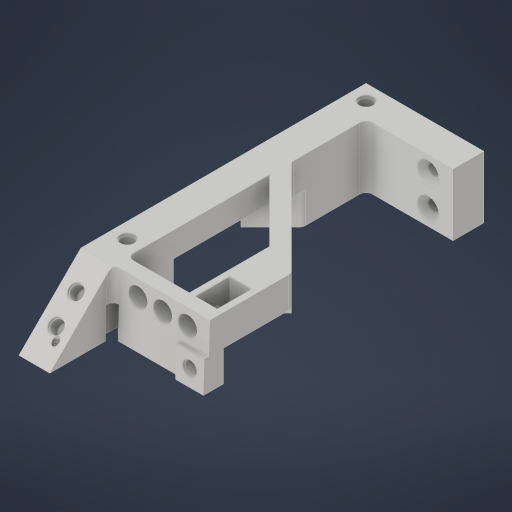
# Autodesk Inventor part: mocowanie-czujnika-p
Saved by Autodesk Inventor 2023 (Build 270158000, 158)
## iProperties
Created: 2019-09-07
Part Number: mocowanie-czujnika-p
Material: Generic
Document SubType Name: Modeling
Designer: Michal
Density: 1 g/cm^3
Appearance: Default
Author: Michal
Autodesk Inventor part; units mm, degrees
note: some values were not read from the file. Chosen so that the rebuilt part matches the saved one: direction of "Hole13".
ref_plane "YZ Plane" through (0, 0, 0) normal (1, 0, 0) x (0, 1, 0)
ref_plane "XZ Plane" through (0, 0, 0) normal (0, 1, 0) x (-1, 0, 0)
sketch "Sketch1" plane through (0, 0, 0) normal (1, 0, 0) x (0, 1, 0)
  line L0 (0, 0) -> (0, 0)
  line L1 (0, 0) -> (0, -3)
  line L2 (0, -3) -> (0, -113)
  line L3 (20, -23) -> (20, -113)
  line L4 (20, -23) -> (20, -20)
  line L5 (20, -20) -> (17, -20)
  line L6 (17, -20) -> (0, -3)
  line L7 (0, -113) -> (0, -115)
  line L8 (0, -115) -> (20, -115)
  line L9 (20, -115) -> (20, -113)
  dimension "d19" = 113
  dimension "d22" = 3
  dimension "d23" = 3
  dimension "d25" = 2
  dimension "d26" = 20
  constraints: 20 end point, 3 vertical, 2 perpendicular, 1 collinear, 1 parallel
  measures "d19" distance of L0.start L2.end
  measures "d22" distance of L0.start L1.end
  measures "d23" distance of L3.start L4.end
  measures "d25" distance of L2.end L7.end
  measures "d26" distance of L7.end L8.end
extrude "Extrusion1" add sketch "Sketch1" along normal blind 10
sketch "Sketch4" plane through (10, 0, 0) normal (1, 0, 0) x (0, 0, -1)
  line L0 (20, 20) -> (115, 20) projected
  line L1 (3, 0) -> (115, 0) projected
  line L2 (115, 20) -> (105, 20)
  line L3 (105, 20) -> (105, 0)
  line L4 (105, 0) -> (115, 0)
  line L5 (115, 0) -> (115, 20)
  point P0 (113, 0)
  dimension "d27" = 10
  constraints: 8 end point, 2 parallel, 1 horizontal, 1 perpendicular, 1 point on line
  measures "d27" distance of L4.end L3.end
extrude "Extrusion4" add sketch "Sketch4" along normal blind 28
sketch "Sketch7" plane through (0, 0, -115) normal (0, -1, 0) x (1, 0, 0)
  line L0 (10, 112) -> (10, 10) projected
  line L1 (10, 112) -> (7, 112)
  line L2 (7, 112) -> (7, 107)
  line L3 (7, 107) -> (10, 107)
  line L4 (10, 107) -> (10, 112)
  point P0 (0, 115)
  dimension "d39" = 3
  dimension "d40" = 5
  constraints: 8 end point, 2 parallel, 1 horizontal, 1 perpendicular
  measures "d39" distance of L3.end L2.end
  measures "d40" distance of L2.end L1.end
hole "Hole2" at (7, 0, -8) direction (0, 1, 0) diameter 2.0066 depth 7.5946
sketch "Sketch8" plane through (0, 0, -115) normal (0, -1, 0) x (1, 0, 0)
  line L0 (0, 0) -> (0, 112) projected
  line L1 (0, 112) -> (5, 112)
  line L2 (5, 112) -> (5, 82)
  line L3 (5, 82) -> (0, 82)
  line L4 (0, 82) -> (0, 112)
  line L5 (0, 0) -> (5, 0)
  line L6 (5, 0) -> (5, 5)
  line L7 (5, 5) -> (0, 5)
  line L8 (0, 5) -> (0, 0)
  line L9 (38, 0) -> (25, 0)
  line L10 (25, 0) -> (25, 5)
  line L11 (25, 5) -> (38, 5)
  line L12 (38, 5) -> (38, 0)
  point P0 (0, 115)
  dimension "d48" = 5
  dimension "d49" = 30
  dimension "d50" = 5
  dimension "d51" = 5
  dimension "d97" = 13
  dimension "d98" = 5
  constraints: 24 end point, 6 parallel, 3 horizontal, 3 perpendicular
  measures "d48" distance of L2.end L3.end
  measures "d49" distance of L1.end L2.end
  measures "d50" distance of L7.end L6.end
  measures "d51" distance of L6.end L5.end
  measures "d97" distance of L10.end L11.end
  measures "d98" distance of L9.end L10.end
hole "Hole3" at (5, 0, -110) at (5, 0, -33) at (25, 0, -110) direction (0, 1, 0) diameter 6 depth 6 counterbore diameter 6.5 counterbore depth 2
sketch "Sketch9" plane through (0, 0, 0) normal (-1, 0, 0) x (0, 0, 1)
  line L0 (-20, 20) -> (-115, 20) projected
  line L1 (-20, 20) -> (-25, 20)
  line L2 (-25, 20) -> (-25, 15)
  line L3 (-25, 15) -> (-20, 15)
  line L4 (-20, 15) -> (-20, 20)
  line L5 (-115, 20) -> (-105, 20)
  line L6 (-105, 20) -> (-105, 15)
  line L7 (-105, 15) -> (-115, 15)
  line L8 (-115, 15) -> (-115, 20)
  line L9 (-115, 20) -> (-115, 0) projected
  line L10 (-115, 0) -> (-105, 0)
  line L11 (-105, 0) -> (-105, 5)
  line L12 (-105, 5) -> (-115, 5)
  line L13 (-115, 5) -> (-115, 0)
  line L14 (-20, 9) -> (-20, 0) projected
  line L15 (-20, 0) -> (-25, 0)
  line L16 (-25, 0) -> (-25, 5)
  line L17 (-25, 5) -> (-20, 5)
  line L18 (-20, 5) -> (-20, 0)
  point P0 (0, 0)
  dimension "d61" = 5
  dimension "d62" = 5
  dimension "d63" = 10
  dimension "d64" = 10
  dimension "d65" = 5
  constraints: 32 end point, 8 parallel, 4 horizontal, 4 perpendicular
  measures "d61" distance of L3.end L2.end
  measures "d62" distance of L2.end L1.end
  measures "d63" distance of L6.end L7.end
  measures "d64" distance of L12.end L11.end
  measures "d65" distance of L11.end L10.end
hole "Hole4" at (0, 15, -105) at (0, 5, -105) at (0, 15, -25) at (0, 5, -25) direction (1, 0, 0) diameter 4 depth 4 counterbore diameter 4.5 counterbore depth 0.6
sketch "Sketch10" plane through (0, 0, -3) normal (0, 0.7071068, 0.7071068) x (1, 0, 0)
  line L0 (0, 0) -> (5, 0)
  line L1 (5, 0) -> (5, 10)
  line L2 (5, 10) -> (0, 10)
  line L3 (0, 10) -> (0, 0)
  line L4 (0, 24.0416) -> (10, 24.0416) projected
  line L5 (0, 24.0416) -> (5, 24.0416)
  line L6 (5, 24.0416) -> (5, 19.0416)
  line L7 (5, 19.0416) -> (0, 19.0416)
  line L8 (0, 19.0416) -> (0, 24.0416)
  dimension "d73" = 5
  dimension "d74" = 10
  dimension "d75" = 5
  dimension "d76" = 5
  constraints: 16 end point, 4 parallel, 2 horizontal, 2 perpendicular
  measures "d73" distance of L2.end L1.end
  measures "d74" distance of L1.end L0.end
  measures "d75" distance of L6.end L7.end
  measures "d76" distance of L5.end L6.end
hole "Hole5" at (5, 13.4645, -16.4645) at (5, 7.0711, -10.0711) direction (0, -0.7071068, -0.7071068) diameter 4 depth 4 counterbore diameter 4.5 counterbore depth 0.6
sketch "Sketch6" plane through (10, 0, -105) normal (0, 0, 1) x (1, 0, 0)
  line L0 (28, 20) -> (28, 0) projected
  line L1 (28, 20) -> (20, 20)
  line L2 (20, 20) -> (20, 15)
  line L3 (20, 15) -> (28, 15)
  line L4 (28, 15) -> (28, 20)
  line L5 (28, 0) -> (20, 0)
  line L6 (20, 0) -> (20, 5)
  line L7 (20, 5) -> (28, 5)
  line L8 (28, 5) -> (28, 0)
  point P0 (-10, 0)
  point P1 (23, 15)
  point P2 (23, 5)
  dimension "d84" = 8
  dimension "d85" = 5
  dimension "d86" = 8
  dimension "d87" = 5
  constraints: 16 end point, 4 parallel, 2 horizontal, 2 perpendicular
  measures "d84" distance of L3.end L2.end
  measures "d85" distance of L2.end L1.end
  measures "d86" distance of L6.end L7.end
  measures "d87" distance of L5.end L6.end
hole "Hole6" at (30, 15, -105) at (30, 5, -105) direction (0, 0, -1) diameter 3.4 end through all countersink diameter 6.9 countersink angle 89.954 clearance for "Countersunk Flat Head Screw ISO 2009/7046" size "M3" standard "ISO"
sketch "Sketch12" plane through (0, 0, 0) normal (-1, 0, 0) x (0, 0, 1)
  line L0 (-20, 17) -> (-3, 0) projected
  line L1 (-20, 17) -> (-20, 20) projected
  line L2 (-20, 17) -> (-20, 20)
  line L3 (-20, 17) -> (-23, 20)
  line L4 (-35, 20) -> (-20, 20) projected
  line L5 (-23, 20) -> (-20, 20)
  point P0 (0, 0)
  constraints: 6 end point, 2 collinear
extrude "Extrusion5" cut sketch "Sketch12" against normal blind 35
sketch "Sketch16" plane through (0, 20, -23) normal (0, 1, 0) x (1, 0, 0)
  circle A0 centre (5, 10) radius 3 projected
  circle A1 centre (5, 87) radius 3 projected
  circle A2 centre (5, 10) radius 1.5
  circle A3 centre (5, 87) radius 1.5
  point P0 (0, -23)
  dimension "d124" = 3
  dimension "d125" = 3
  constraints: 2 centre point, 2 coincident
  measures "d124" diameter of A2
  measures "d125" diameter of A3
hole "Hole11" at (5, 20, -110) at (5, 20, -33) direction (0, -1, 0) diameter 4 depth 4 counterbore diameter 4.5 counterbore depth 0.6
sketch "Sketch35" plane through (10, 0, 0) normal (1, 0, 0) x (0, 0, -1)
  line L0 (105, 20) -> (23, 20) projected
  line L1 (3, 0) -> (23, 20)
  line L2 (23, 20) -> (28, 20)
  line L3 (28, 20) -> (28, 0)
  line L4 (28, 0) -> (3, 0)
  point P0 (0, 0)
  dimension "d247" = 5
  constraints: 8 end point, 2 perpendicular, 1 point on line
  measures "d247" distance of L0.end L2.end
extrude "Extrusion22" add sketch "Sketch35" along normal blind 34
sketch "Sketch36" plane through (0, 0, -115) normal (0, -1, 0) x (1, 0, 0)
  line L0 (0, 112) -> (44, 112) projected
  line L1 (44, 112) -> (10, 112)
  line L2 (10, 112) -> (10, 92)
  line L3 (10, 92) -> (44, 92)
  line L4 (44, 92) -> (44, 112)
  line L5 (10, 87) -> (44, 87) projected
  line L6 (44, 92) -> (41, 92)
  line L7 (41, 92) -> (41, 87)
  line L8 (41, 87) -> (44, 87)
  line L9 (44, 87) -> (44, 92)
  point P0 (0, 115)
  dimension "d250" = 34
  dimension "d251" = 20
  dimension "d270" = 3
  constraints: 16 end point, 4 parallel, 2 horizontal, 2 perpendicular, 1 point on line
  measures "d250" distance of L3.end L2.end
  measures "d251" distance of L2.end L1.end
  measures "d270" distance of L8.end L7.end
extrude "Extrusion23" cut sketch "Sketch36" against normal up to next
chamfer "Chamfer3" distance 20 angle 1.72 1 edges at (25.5, 20, -23) measured on face at (20.3333, 6.6667, -23)
sketch "Sketch37" plane through (0, 0, -115) normal (0, -1, 0) x (1, 0, 0)
  line L0 (0, 84.0724) -> (16.2635, 67.809)
  line L1 (0, 84.0724) -> (23, 84.0724) construction
  circle A0 centre (5, 82) radius 2.0701 projected
  line L2 (0, 0) -> (0, 112) projected
  line L3 (0, 84.0724) -> (0, 82.0724)
  line L4 (0, 82.0724) -> (18.3848, 63.6877)
  line L5 (18.3848, 63.6877) -> (0, 45.3029)
  line L6 (0, 45.3029) -> (4.9497, 40.3531)
  line L7 (4.9497, 40.3531) -> (2.4749, 37.8783)
  line L8 (2.4749, 37.8783) -> (4.5962, 35.7569)
  line L9 (4.5962, 35.7569) -> (25.4558, 56.6166)
  line L10 (25.4558, 56.6166) -> (18.3848, 63.6877)
  line L11 (0, 82.0724) -> (0, 45.3029)
  line L12 (2.4749, 37.8783) -> (0, 40.3531)
  line L13 (0, 45.3029) -> (0, 40.3531)
  point P0 (0, 115)
  dimension "d258" = 45
  dimension "d259" = 2
  dimension "d260" = 26
  dimension "d261" = 7
  dimension "d262" = 3.5
  dimension "d263" = 3
  constraints: 26 end point, 6 perpendicular, 5 point on line, 1 collinear, 1 equal length, 1 horizontal, 1 parallel, 1 tangent
  measures "d258" angle of L0 L1
  measures "d259" distance of L0.start L3.end
  measures "d260" distance of L3.end L4.end
  measures "d261" distance of L5.end L6.end
  measures "d262" distance of L6.end L7.end
  measures "d263" distance of L7.end L8.end
extrude "Extrusion24" cut sketch "Sketch37" against normal blind 12 contours L2 L6 L7 L12 | L2 L4 L5 | L5 L10 L9 L8 L7 L6
sketch "Sketch38" plane through (0, 0, -115) normal (0, -1, 0) x (1, 0, 0)
  line L0 (10, 41.1607) -> (4.5962, 35.7569) projected
  line L1 (4.5962, 35.7569) -> (28.6378, 59.7986)
  line L2 (28.6378, 59.7986) -> (32.1734, 56.263)
  line L3 (32.1734, 56.263) -> (8.1317, 32.2214)
  line L4 (8.1317, 32.2214) -> (4.5962, 35.7569)
  point P0 (0, 115)
  dimension "d266" = 34
  dimension "d267" = 5
  constraints: 8 end point, 2 perpendicular, 1 collinear, 1 parallel
  measures "d266" distance of L0.end L1.end
  measures "d267" distance of L1.end L2.end
extrude "Extrusion25" add sketch "Sketch38" against normal blind 20
sketch "Sketch39" plane through (4.5962, 0, -79.2431) normal (-0.7071068, 0, 0.7071068) x (0.7071068, 0, 0.7071068)
  line L0 (0, 0) -> (0, 12) projected
  line L1 (0, 0) -> (0, 10)
  line L2 (0, 0) -> (10, 0)
  line L3 (2.6421, 0) -> (-14.3918, 0) projected
  line L4 (10, 0) -> (10, 10)
  line L5 (0, 10) -> (10, 10)
  line L6 (2.6421, 20) -> (2.6421, 0) projected
  point P0 (52.7833, 0)
  dimension "d271" = 10
  dimension "d272" = 10
  constraints: 8 end point, 1 collinear, 1 parallel, 1 perpendicular, 1 point on line
  measures "d271" distance of L0.start L1.end
  measures "d272" distance of L0.start L2.end
extrude "Extrusion26" cut sketch "Sketch39" against normal up to next
sketch "Sketch43" plane through (0, 20, -23) normal (0, 1, 0) x (1, 0, 0)
  line L0 (41, 5) -> (41, 18)
  line L1 (41, 18) -> (30, 18)
  line L2 (30, 18) -> (30, 5)
  line L3 (32.1734, 35.737) -> (15.2028, 52.7075) construction
  line L4 (10, 50.8393) -> (28.6378, 32.2014) construction
  line L5 (32.1734, 35.737) -> (28.6378, 32.2014)
  line L6 (28.6378, 32.2014) -> (32.1734, 35.737) projected
  line L7 (28.6378, 32.2014) -> (30, 30.8393)
  line L8 (30, 30.8393) -> (30, 18)
  line L9 (32.1734, 35.737) -> (41, 26.9103)
  line L10 (41, 26.9103) -> (41, 18)
  line L11 (41, 5) -> (30, 5)
  line L12 (10, 5) -> (41, 5) projected
  point P0 (0, -23)
  dimension "d297" = 13
  dimension "d298" = 11
  constraints: 18 end point, 4 perpendicular, 4 vertical, 2 point on line, 1 collinear
  measures "d297" distance of L0.start L0.end
  measures "d298" distance of L0.end L1.end
extrude "Extrusion28" add sketch "Sketch43" against normal blind 10
sketch "Sketch44" plane through (0, 20, -23) normal (0, 1, 0) x (1, 0, 0)
  line L0 (30, 5) -> (30, 30.8393) construction
  line L1 (30, 5) -> (32, 5) construction
  line L2 (10, 5) -> (41, 5) construction
  line L3 (32, 5) -> (39, 5)
  line L4 (39, 5) -> (39, 16)
  line L5 (39, 16) -> (32, 16)
  line L6 (32, 16) -> (32, 5)
  point P0 (0, -23)
  point P1 (15, 5)
  dimension "d301" = 2
  dimension "d302" = 7
  dimension "d303" = 11
  constraints: 10 end point, 2 parallel, 1 horizontal, 1 perpendicular, 1 point on line
  measures "d301" distance of L0.start L1.end
  measures "d302" distance of L5.end L4.end
  measures "d303" distance of L4.end L3.end
extrude "Extrusion29" cut sketch "Sketch44" against normal up to next
sketch "Sketch45" plane through (32, 20, -28) normal (1, 0, 0) x (0, 0, -1)
  line L0 (0, 0) -> (0, -10) construction
  line L1 (0, -10) -> (4, -10) construction
  line L2 (11, -10) -> (0, -10) construction
  line L3 (4, -10) -> (7, -10)
  line L4 (7, -10) -> (7, -6)
  line L5 (7, -6) -> (4, -6)
  line L6 (4, -6) -> (4, -10)
  point P0 (-28, -20)
  dimension "d306" = 4
  dimension "d307" = 3
  dimension "d308" = 4
  constraints: 10 end point, 2 parallel, 1 horizontal, 1 perpendicular, 1 point on line
  measures "d306" distance of L0.end L1.end
  measures "d307" distance of L5.end L4.end
  measures "d308" distance of L4.end L3.end
extrude "Extrusion30" add sketch "Sketch45" along normal up to next
sketch "Sketch46" plane through (15.2028, 0, -75.7075) normal (0.7071068, 0, -0.7071068) x (-0.7071068, 0, -0.7071068)
  line L0 (7.3579, 20) -> (7.3579, 10) construction
  line L1 (7.3579, 20) -> (7.3579, 15) construction
  line L2 (7.3579, 15) -> (-2.6421, 15) construction
  line L3 (-2.6421, 15) -> (-10.6421, 15) construction
  line L4 (-10.6421, 15) -> (-18.6421, 15) construction
  line L5 (-18.6421, 15) -> (-26.6421, 15) construction
  circle A0 centre (-2.6421, 15) radius 3
  circle A1 centre (-10.6421, 15) radius 3
  circle A2 centre (-18.6421, 15) radius 3
  circle A3 centre (-26.6421, 15) radius 3
  point P0 (-42.7833, 0)
  dimension "d311" = 5
  dimension "d312" = 10
  dimension "d313" = 8
  dimension "d314" = 8
  dimension "d315" = 8
  dimension "d316" = 6
  dimension "d317" = 6
  dimension "d318" = 6
  dimension "d319" = 6
  constraints: 10 end point, 4 centre point, 4 coincident, 3 horizontal, 1 midpoint, 1 point on line
  measures "d311" distance of L0.start L1.end
  measures "d312" distance of L1.end L2.end
  measures "d313" distance of L2.end L3.end
  measures "d314" distance of L3.end L4.end
  measures "d315" distance of L4.end L5.end
  measures "d316" diameter of A0
  measures "d317" diameter of A1
  measures "d318" diameter of A2
  measures "d319" diameter of A3
extrude "Extrusion31" cut sketch "Sketch46" against normal up to next
ref_plane "Work Plane4" through (10, 9.8544, -28) normal (0, 0, -1) x (-1, 0, 0)
sketch "Sketch47" plane through (10, 9.8544, -28) normal (0, 0, -1) x (-1, 0, 0)
  line L0 (0, 10.1456) -> (0, 5.1456) construction
  line L1 (0, 5.1456) -> (-8, 5.1456) construction
  line L2 (-8, 5.1456) -> (-16, 5.1456) construction
  line L3 (-16, 5.1456) -> (-24, 5.1456) construction
  circle A0 centre (-24, 5.1456) radius 3
  circle A1 centre (-16, 5.1456) radius 3
  circle A2 centre (-8, 5.1456) radius 3
  point P0 (10, -9.8544)
  dimension "d322" = 5
  dimension "d323" = 8
  dimension "d324" = 8
  dimension "d325" = 8
  dimension "d326" = 6
  dimension "d327" = 6
  dimension "d328" = 6
  constraints: 8 end point, 3 centre point, 3 coincident, 2 point on line, 1 horizontal, 1 vertical
  measures "d322" distance of L0.start L0.end
  measures "d323" distance of L0.end L1.end
  measures "d324" distance of L1.end L2.end
  measures "d325" distance of L2.end L3.end
  measures "d326" diameter of A0
  measures "d327" diameter of A1
  measures "d328" diameter of A2
extrude "Extrusion32" cut sketch "Sketch47" against normal up to next
sketch "Sketch48" plane through (10, 0, 0) normal (1, 0, 0) x (0, 0, -1)
  line L0 (28, 0) -> (28, 9.8544) projected
  line L1 (28, 0) -> (21, 0)
  line L2 (21, 0) -> (21, 10)
  line L3 (21, 10) -> (28, 10)
  line L4 (28, 10) -> (28, 0)
  point P0 (0, 0)
  dimension "d331" = 7
  dimension "d332" = 10
  constraints: 8 end point, 2 parallel, 1 horizontal, 1 perpendicular
  measures "d331" distance of L2.end L3.end
  measures "d332" distance of L1.end L2.end
extrude "Extrusion33" cut sketch "Sketch48" along normal mid plane 4
sketch "Sketch49" plane through (0, 0, -3) normal (0, -1, 0) x (1, 0, 0)
  line L0 (10, -25) -> (8, -25) projected
  line L1 (10, -70.8393) -> (10, -25) projected
  line L2 (8, -25) -> (10, -25)
  line L3 (10, -25) -> (10, -27)
  line L4 (10, -27) -> (8, -25)
  point P0 (0, 3)
  dimension "d335" = 2
  constraints: 6 end point, 1 perpendicular, 1 point on line
  measures "d335" distance of L0.start L3.end
extrude "Extrusion34" cut sketch "Sketch49" against normal blind 10
sketch "Sketch50" plane through (10, 20, -23.6006) normal (0, 0.0300152, 0.9995494) x (1, 0, 0)
  line L0 (31, -20.009) -> (31, 0) projected
  line L1 (31, -20.009) -> (22, -20.009)
  line L2 (22, -20.009) -> (22, -10.009)
  line L3 (22, -10.009) -> (31, -10.009)
  line L4 (31, -10.009) -> (31, -20.009)
  point P0 (-10, -20.6994)
  dimension "d338" = 10
  dimension "d339" = 9
  constraints: 8 end point, 2 parallel, 1 horizontal, 1 perpendicular
  measures "d338" distance of L1.end L2.end
  measures "d339" distance of L2.end L3.end
extrude "Extrusion35" add sketch "Sketch50" along normal blind 1.5
sketch "Sketch51" plane through (10, 12, -73.8393) normal (-0.7071068, 0, 0.7071068) x (0.7071068, 0, 0.7071068)
  line L0 (26.3579, -12) -> (2.3579, -12) projected
  line L1 (26.3579, -12) -> (17.3579, -12)
  line L2 (17.3579, -12) -> (17.3579, -2)
  line L3 (17.3579, -2) -> (26.3579, -2)
  line L4 (26.3579, -2) -> (26.3579, -12)
  point P0 (45.1412, -12)
  dimension "d342" = 9
  dimension "d343" = 10
  constraints: 8 end point, 2 parallel, 1 horizontal, 1 perpendicular
  measures "d342" distance of L2.end L3.end
  measures "d343" distance of L1.end L2.end
extrude "Extrusion36" add sketch "Sketch51" along normal blind 1.5
sketch "Sketch42" plane through (32.1734, 0, -58.737) normal (0.7071068, 0, -0.7071068) x (-0.7071068, 0, -0.7071068)
  line L0 (0, 0) -> (0, 20) projected
  line L1 (0, 0) -> (4.5, 0)
  line L2 (4.5, 0) -> (4.5, 5.25)
  line L3 (4.5, 5.25) -> (0, 5.25)
  line L4 (0, 5.25) -> (0, 0)
  point P0 (-18.7833, 0)
  dimension "d288" = 4.5
  dimension "d289" = 5.25
  constraints: 8 end point, 2 parallel, 1 horizontal, 1 perpendicular
  measures "d288" distance of L3.end L2.end
  measures "d289" distance of L2.end L1.end
hole "Hole13" at (28.9914, 5.25, -61.9189) direction (-0.7071068, 0, 0.7071068) diameter 3.4 depth 6.5 countersink diameter 6.9 countersink angle 89.954 clearance for "Countersunk Flat Head Screw ISO 2009/7046" size "M3" standard "ISO"
sketch "Sketch41" plane through (10, 20.045, -22.1012) normal (0, 0.0300152, 0.9995494) x (1, 0, 0)
  line L0 (31, -19.8589) -> (31, -20.009) projected
  line L1 (31, -20.009) -> (26.5, -20.009)
  line L2 (26.5, -20.009) -> (26.5, -14.759)
  line L3 (26.5, -14.759) -> (31, -14.759)
  line L4 (31, -14.759) -> (31, -20.009)
  point P0 (-10, -20.6994)
  dimension "d279" = 4.5
  dimension "d280" = 5.25
  constraints: 8 end point, 2 parallel, 1 horizontal, 1 perpendicular
  measures "d279" distance of L2.end L3.end
  measures "d280" distance of L1.end L2.end
hole "Hole12" at (36.5, 5.2927, -21.6583) direction (0, -0.0300152, -0.9995494) diameter 4 depth 4 counterbore diameter 4.5 counterbore depth 0.6
fillet "Fillet1" radius 2 6 edges at (10, 15, -28) (10, 15, -23.4504) (10, 15, -80.9103) (10, 10, -105) (10, 5, -84.6469) (41, 15, -49.9103)
body "Solid1"
